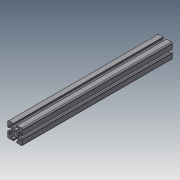
# Autodesk Inventor part: 5537T709.step
Saved by Autodesk Inventor 2018.3 (Build 223284000, 284)
## iProperties
Created: 2015-02-25
Material: Generic
Vendor: HHMI: JRC - ID&F
Document SubType Name: Modeling
Designer: arnoldj
Density: 1 g/cm^3
Appearance: Default
RuleStatus: InUse
AfterDocSave0: file://Part Number Cleaner
DESIGN DEPARTMENT: HHMI: JRC - ID&F
ALTERED ITEM PART NUMBER: N/A
ALTERED ITEM VENDOR: N/A
ALTERED ITEM DESCRIPTION: N/A
Revision: ANY
Title: 5537T709.step
Description: STEP AP203
Sending System: SolidWorks 2010
Preprocessor: SwSTEP 2.0
Author: arnoldj
Revision Number: 0
Autodesk Inventor part; units mm, degrees
ref_plane "YZ Plane" through (0, 0, 0) normal (1, 0, 0) x (0, 1, 0)
ref_plane "XZ Plane" through (0, 0, 0) normal (0, 1, 0) x (-1, 0, 0)
ref_plane "XY Plane" through (0, 0, 0) normal (0, 0, 1) x (1, 0, 0)
sketch "Sketch1" plane through (-16.952, 20, 0) normal (0, 0, 1) x (1, 0, 0)
  arc A0 (11.758, -11.3649) -> (13.8774, -12.2428) centre (13.8774, -9.2456) ccw projected
  line L0 (11.758, -11.3649) -> (6.1897, -5.7966) projected
  arc A1 (6.7285, -4.4958) -> (6.1897, -5.7966) centre (6.7285, -5.2578) ccw projected
  line L1 (6.7285, -4.4958) -> (12.1895, -4.4958) projected
  arc A2 (12.1895, -4.4958) -> (12.9515, -3.7338) centre (12.1895, -3.7338) ccw projected
  line L2 (12.9515, -3.7338) -> (12.9515, -0.762) projected
  arc A3 (12.9515, -0.762) -> (12.1895, 0) centre (12.1895, -0.762) ccw projected
  line L3 (12.1895, 0) -> (0, 0) projected
  arc A4 (0, 0) -> (-3.048, -3.048) centre (0, -3.048) ccw projected
  line L4 (-3.048, -3.048) -> (-3.048, -15.2375) projected
  arc A5 (-3.048, -15.2375) -> (-2.286, -15.9995) centre (-2.286, -15.2375) ccw projected
  line L5 (-2.286, -15.9995) -> (0.6858, -15.9995) projected
  arc A6 (0.6858, -15.9995) -> (1.4478, -15.2375) centre (0.6858, -15.2375) ccw projected
  line L6 (1.4478, -15.2375) -> (1.4478, -9.7765) projected
  arc A7 (2.7486, -9.2377) -> (1.4478, -9.7765) centre (2.2098, -9.7765) ccw projected
  line L7 (2.7486, -9.2377) -> (8.3169, -14.806) projected
  arc A8 (9.1948, -16.9254) -> (8.3169, -14.806) centre (6.1976, -16.9254) ccw projected
  line L8 (9.1948, -16.9254) -> (9.1948, -23.0746) projected
  arc A9 (8.3169, -25.194) -> (9.1948, -23.0746) centre (6.1976, -23.0746) ccw projected
  line L9 (8.3169, -25.194) -> (2.7486, -30.7623) projected
  arc A10 (1.4478, -30.2235) -> (2.7486, -30.7623) centre (2.2098, -30.2235) ccw projected
  line L10 (1.4478, -30.2235) -> (1.4478, -24.7625) projected
  arc A11 (1.4478, -24.7625) -> (0.6858, -24.0005) centre (0.6858, -24.7625) ccw projected
  line L11 (0.6858, -24.0005) -> (-2.286, -24.0005) projected
  arc A12 (-2.286, -24.0005) -> (-3.048, -24.7625) centre (-2.286, -24.7625) ccw projected
  line L12 (-3.048, -24.7625) -> (-3.048, -36.952) projected
  arc A13 (-3.048, -36.952) -> (0, -40) centre (0, -36.952) ccw projected
  line L13 (0, -40) -> (12.1895, -40) projected
  arc A14 (12.1895, -40) -> (12.9515, -39.238) centre (12.1895, -39.238) ccw projected
  line L14 (12.9515, -39.238) -> (12.9515, -36.2662) projected
  arc A15 (12.9515, -36.2662) -> (12.1895, -35.5042) centre (12.1895, -36.2662) ccw projected
  line L15 (12.1895, -35.5042) -> (6.7285, -35.5042) projected
  arc A16 (6.1897, -34.2034) -> (6.7285, -35.5042) centre (6.7285, -34.7422) ccw projected
  line L16 (6.1897, -34.2034) -> (11.758, -28.6351) projected
  arc A17 (13.8774, -27.7572) -> (11.758, -28.6351) centre (13.8774, -30.7544) ccw projected
  line L17 (13.8774, -27.7572) -> (20.0266, -27.7572) projected
  arc A18 (22.146, -28.6351) -> (20.0266, -27.7572) centre (20.0266, -30.7544) ccw projected
  line L18 (22.146, -28.6351) -> (27.7143, -34.2034) projected
  arc A19 (27.1755, -35.5042) -> (27.7143, -34.2034) centre (27.1755, -34.7422) ccw projected
  line L19 (27.1755, -35.5042) -> (21.7145, -35.5042) projected
  arc A20 (21.7145, -35.5042) -> (20.9525, -36.2662) centre (21.7145, -36.2662) ccw projected
  line L20 (20.9525, -36.2662) -> (20.9525, -39.238) projected
  arc A21 (20.9525, -39.238) -> (21.7145, -40) centre (21.7145, -39.238) ccw projected
  line L21 (21.7145, -40) -> (33.904, -40) projected
  arc A22 (33.904, -40) -> (36.952, -36.952) centre (33.904, -36.952) ccw projected
  line L22 (36.952, -36.952) -> (36.952, -24.7625) projected
  arc A23 (36.952, -24.7625) -> (36.19, -24.0005) centre (36.19, -24.7625) ccw projected
  line L23 (36.19, -24.0005) -> (33.2182, -24.0005) projected
  arc A24 (33.2182, -24.0005) -> (32.4562, -24.7625) centre (33.2182, -24.7625) ccw projected
  line L24 (32.4562, -24.7625) -> (32.4562, -30.2235) projected
  arc A25 (31.1554, -30.7623) -> (32.4562, -30.2235) centre (31.6942, -30.2235) ccw projected
  line L25 (31.1554, -30.7623) -> (25.5871, -25.194) projected
  arc A26 (24.7092, -23.0746) -> (25.5871, -25.194) centre (27.7064, -23.0746) ccw projected
  line L26 (24.7092, -23.0746) -> (24.7092, -16.9254) projected
  arc A27 (25.5871, -14.806) -> (24.7092, -16.9254) centre (27.7064, -16.9254) ccw projected
  line L27 (25.5871, -14.806) -> (31.1554, -9.2377) projected
  arc A28 (32.4562, -9.7765) -> (31.1554, -9.2377) centre (31.6942, -9.7765) ccw projected
  line L28 (32.4562, -9.7765) -> (32.4562, -15.2375) projected
  arc A29 (32.4562, -15.2375) -> (33.2182, -15.9995) centre (33.2182, -15.2375) ccw projected
  line L29 (33.2182, -15.9995) -> (36.19, -15.9995) projected
  arc A30 (36.19, -15.9995) -> (36.952, -15.2375) centre (36.19, -15.2375) ccw projected
  line L30 (36.952, -15.2375) -> (36.952, -3.048) projected
  arc A31 (36.952, -3.048) -> (33.904, 0) centre (33.904, -3.048) ccw projected
  line L31 (33.904, 0) -> (21.7145, 0) projected
  arc A32 (21.7145, 0) -> (20.9525, -0.762) centre (21.7145, -0.762) ccw projected
  line L32 (20.9525, -0.762) -> (20.9525, -3.7338) projected
  arc A33 (20.9525, -3.7338) -> (21.7145, -4.4958) centre (21.7145, -3.7338) ccw projected
  line L33 (21.7145, -4.4958) -> (27.1755, -4.4958) projected
  arc A34 (27.7143, -5.7966) -> (27.1755, -4.4958) centre (27.1755, -5.2578) ccw projected
  line L34 (27.7143, -5.7966) -> (22.146, -11.3649) projected
  arc A35 (20.0266, -12.2428) -> (22.146, -11.3649) centre (20.0266, -9.2456) ccw projected
  line L35 (20.0266, -12.2428) -> (13.8774, -12.2428) projected
  circle A36 centre (16.952, -20) radius 3.4036 projected
extrude "Extrusion1" add sketch "Sketch1" along normal mid plane 394.335
body "Solid2"
